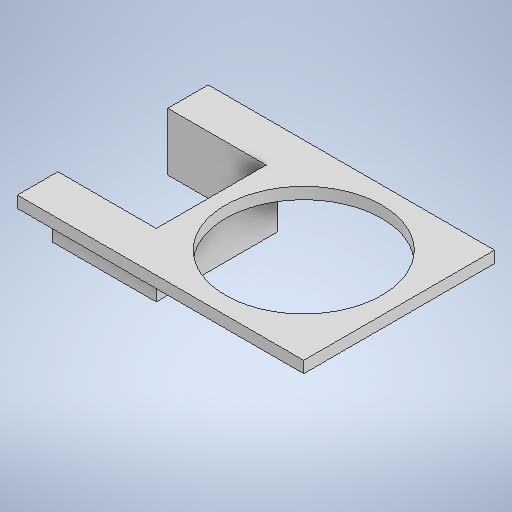
# Autodesk Inventor part: joystick_test_v2
Saved by Autodesk Inventor 2025.4 (Build 294407000, 407)
## iProperties
Created: 2026-07-26
Part Number: joystick_test_v2
Material: Generic
Document SubType Name: Modeling
Designer: Franchesca
Density: 1 g/cm^3
Appearance: Default
Author: Franchesca
Autodesk Inventor part; units mm, degrees
ref_plane "YZ Plane" through (0, 0, 0) normal (1, 0, 0) x (0, 1, 0)
ref_plane "XZ Plane" through (0, 0, 0) normal (0, 1, 0) x (-1, 0, 0)
ref_plane "XY Plane" through (0, 0, 0) normal (0, 0, 1) x (1, 0, 0)
sketch "Sketch1" plane through (0, 0, 0) normal (0, 1, 0) x (-1, 0, 0)
  circle A0 centre (0, 0) radius 13.5
  line L0 (0, -13.5) -> (30, -13.5) construction
  line L1 (0, 13.5) -> (30, 13.5) construction
  line L2 (30, 13.5) -> (30, -13.5) construction
  line L3 (0, -13.5) -> (16, -13.5) construction
  line L4 (0, 13.5) -> (16, 13.5) construction
  line L5 (16, 13.5) -> (16, -13.5) construction
  line L6 (30, 13.5) -> (30, 9.5) construction
  line L7 (30, -13.5) -> (30, -9.5) construction
  line L8 (30, 9.5) -> (16, 9.5)
  line L9 (30, -9.5) -> (16, -9.5)
  line L10 (16, -9.5) -> (16, 9.5)
  line L11 (0, -13.5) -> (0, -16.5) construction
  line L12 (0, 13.5) -> (0, 16.5) construction
  line L13 (30, -2.5) -> (33, -2.5) construction
  line L14 (-13.5, 0) -> (-16.5, 0) construction
  line L15 (33, -2.5) -> (33, -16.5)
  line L16 (33, -16.5) -> (0, -16.5)
  line L17 (33, -2.5) -> (33, 16.5)
  line L18 (33, 16.5) -> (0, 16.5)
  line L19 (0, 16.5) -> (-16.5, 16.5)
  line L20 (-16.5, 0) -> (-16.5, 16.5)
  line L21 (0, -16.5) -> (-16.5, -16.5)
  line L22 (-16.5, -16.5) -> (-16.5, 0)
  line L23 (30, 9.5) -> (33, 9.5)
  line L24 (30, -9.5) -> (33, -9.5)
  line L25 (0, 13.5) -> (15, 13.5) construction
  line L26 (0, -13.5) -> (15, -13.5) construction
  line L27 (15, 13.5) -> (15, -13.5) construction
  line L28 (33, 9.5) -> (33, 10.5) construction
  line L29 (33, 10.5) -> (15, 10.5) construction
  line L30 (33, -9.5) -> (33, -10.5) construction
  line L31 (33, -10.5) -> (15, -10.5) construction
  line L32 (15, 10.5) -> (15, -10.5)
  line L33 (15, -10.5) -> (33, -10.5)
  line L34 (15, 10.5) -> (33, 10.5)
  dimension "d0" = 27
  dimension "d1" = 30
  dimension "d2" = 30
  dimension "d3" = 16
  dimension "d4" = 16
  dimension "d5" = 4
  dimension "d6" = 4
  dimension "d7" = 3
  dimension "d8" = 3
  dimension "d9" = 3
  dimension "d10" = 3
  dimension "d15" = 19
  dimension "d16" = 15
  dimension "d17" = 15
  dimension "d18" = 1
  dimension "d19" = 1
  constraints: 70 end point, 16 point on line, 9 perpendicular, 4 collinear, 4 horizontal, 4 vertical, 3 point on circle, 2 tangent, 1 centre point, 1 coincident, 1 midpoint, 1 parallel
  measures "d0" diameter of A0
  measures "d1" distance of L0.start L0.end
  measures "d2" distance of L1.start L1.end
  measures "d3" distance of L0.start L3.end
  measures "d4" distance of L1.start L4.end
  measures "d5" distance of L1.end L6.end
  measures "d6" distance of L0.end L7.end
  measures "d7" distance of L0.start L11.end
  measures "d8" distance of L1.start L12.end
  measures "d9" distance of L13.start L13.end
  measures "d10" distance of L14.start L14.end
  measures "d15" distance between parallel lines of L9 L8
  measures "d16" distance of L1.start L25.end
  measures "d17" distance of L0.start L26.end
  measures "d18" distance of L23.end L28.end
  measures "d19" distance of L24.end L30.end
extrude "Extrusion3" add sketch "Sketch1" against normal blind 2 contours L34 L32 L33 L15 L16 L21 L22 L20 L19 L18 L17
extrude "Extrusion4" add sketch "Sketch1" against normal blind 10 contours L8 L10 L9 L24 L15 L33 L32 L34 L17 L23
body "Solid2"
